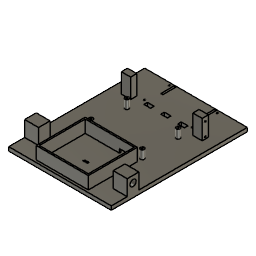
chassis (Autodesk Fusion 360 design; units mm, degrees)
part number: 2026-04-02-12-57-44-250
Autodesk Fusion 360 part; units mm, degrees
other "DerivedContext1"
sketch "Sketch1" plane through (0, 0, 0) normal (0, 0, 1) x (1, 0, 0)
  line L0 (0, 0) -> (132, 0)
  line L1 (132, 0) -> (132, 175)
  line L2 (132, 175) -> (0, 175)
  line L3 (0, 175) -> (0, 0)
  dimension "d1" = 132
  dimension "d2" = 175
  constraint horizontal L0
  constraint horizontal L2
  constraint coincident L0.start L3.end
  measures "d1" distance of L0.start L0.end
  measures "d2" distance of L0.end L1.end
extrude "Extrude1" add sketch "Sketch1" along normal blind 5
sketch "Sketch2" plane through (0, 0, 5) normal (0, 0, 1) x (-1, 0, 0)
  line L0 (0, -175) -> (0, 0)
  line L1 (0, 0) -> (-132, 0)
  line L2 (-132, 0) -> (-132, -175)
  line L3 (-132, -175) -> (0, -175)
  line L4 (-14, -175) -> (-14, -134.884) construction
  line L5 (-14, -134.884) -> (0, -134.884) construction
  line L6 (-14, -138.884) -> (-14, -130.884)
  line L7 (-14, -138.884) -> (-26, -138.884)
  line L8 (-26, -138.884) -> (-26, -130.884)
  line L9 (-14, -130.884) -> (-14, -138.884)
  line L10 (-14, -130.884) -> (-26, -130.884)
  line L11 (-66, -175) -> (-66, -165)
  line L12 (-118, -138.884) -> (-106, -138.884)
  line L13 (-106, -138.884) -> (-106, -130.884)
  line L14 (-118, -130.884) -> (-106, -130.884)
  line L15 (-118, -138.884) -> (-118, -130.884)
  dimension "d5" = 40.116
  dimension "d7" = 14
  dimension "d8" = 8
  dimension "d9" = 12
  dimension "d10" = 10
  constraint vertical L4
  constraint coincident L3 L4.start
  constraint coincident L0 L5.end
  constraint perpendicular L0 L5
  constraint vertical L6
  constraint midpoint L4.end L6
  constraint horizontal L7
  constraint vertical L8
  constraint vertical L9
  constraint perpendicular L8 L10
  constraint midpoint L3 L11.start
  constraint perpendicular L3 L11
  constraint symmetric L6.start L11 L12.start
  constraint symmetric L6.end L11 L14.start
  constraint symmetric L7.end L11 L12.end
  constraint symmetric L8.end L11 L13.end
  measures "d5" distance of L4.start L4.end
  measures "d7" distance of L4.end L5.end
  measures "d8" distance of L6.start L6.end
  measures "d9" distance of L6.start L7.end
  measures "d10" distance of L11.start L11.end
extrude "Extrude2" add sketch "Sketch2" along normal blind 25 contours L6 L7 L8 L9 L10 | L12 L13 L14 L15
ref_plane "WorkPlane1" through (66, 134.884, 17.5) normal (1, 0, 0) x (0, 1, 0)
sketch "Sketch4" plane through (0, 0, 5) normal (0, 0, 1) x (-1, 0, 0)
  line L0 (-106, -138.884) -> (-118, -138.884)
  line L1 (-118, -138.884) -> (-118, -130.884)
  line L2 (-118, -130.884) -> (-106, -130.884)
  line L3 (-106, -130.884) -> (-106, -138.884)
  line L4 (-14, -138.884) -> (-26, -138.884)
  line L5 (-26, -138.884) -> (-26, -130.884)
  line L6 (-26, -130.884) -> (-14, -130.884)
  line L7 (-14, -130.884) -> (-14, -138.884)
  line L8 (0, -175) -> (0, 0)
  line L9 (0, 0) -> (-132, 0)
  line L10 (-132, 0) -> (-132, -175)
  line L11 (-132, -175) -> (0, -175)
  line L12 (-41.25, -175) -> (-41.25, -157)
  line L13 (-41.25, -157) -> (-38.75, -157)
  line L14 (-38.75, -157) -> (-38.75, -175)
  dimension "d27" = 18
  dimension "d28" = 41.25
  dimension "d29" = 2.5
  constraint coincident L11 L12.start
  constraint perpendicular L11 L12
  constraint perpendicular L12 L13
  constraint vertical L14
  constraint coincident L11 L14.end
  measures "d27" distance of L12.start L12.end
  measures "d28" distance of L8 L12
  measures "d29" distance of L12.end L13.end
extrude "Extrude4" cut sketch "Sketch4" against normal blind 4 contours L11 L12 L13 L14
fillet "Fillet1" radius 4 1 edges at (40, 157, 1)
sketch "Sketch5" plane through (41.25, 0, 0) normal (-1, 0, 0) x (0, -1, 0)
  arc A0 (-161, 1) -> (-157, 5) centre (-161, 5) ccw
  line L0 (-157, 5) -> (-175, 5)
  line L1 (-175, 5) -> (-175, 1)
  line L2 (-175, 1) -> (-161, 1)
  line L3 (-175, 5) -> (-171, 5)
  circle A1 centre (-171, 5) radius 4
  dimension "d34" = 4
  dimension "d35" = 8
  constraint coincident L0.end L1.start
  constraint perpendicular L1 L3
  constraint coincident L3.end A1.centre
  measures "d34" distance of L0.end L3.end
  measures "d35" diameter of A1
extrude "Extrude5" add sketch "Sketch5" along normal blind 3 contours L1 L2 A1
ref_plane "WorkPlane3" through (66, 87.5, 2.5) normal (1, 0, 0) x (0, 1, 0)
mirror "Mirror2" about plane through (66, 87.5, 2.5) normal (1, 0, 0) of "Extrude4", "Fillet1", "Extrude5"
sketch "Battery Holder slot" plane through (0, 0, 5) normal (0, 0, 1) x (-1, 0, 0)
  line L0 (-14, -138.884) -> (-26, -138.884)
  line L1 (-26, -138.884) -> (-26, -130.884)
  line L2 (-26, -130.884) -> (-14, -130.884)
  line L3 (-14, -130.884) -> (-14, -138.884)
  line L4 (-106, -138.884) -> (-118, -138.884)
  line L5 (-118, -138.884) -> (-118, -130.884)
  line L6 (-118, -130.884) -> (-106, -130.884)
  line L7 (-106, -130.884) -> (-106, -138.884)
  line L8 (-93.25, -175) -> (-93.25, -157)
  line L9 (-93.25, -157) -> (-90.75, -157)
  line L10 (-90.75, -157) -> (-90.75, -175)
  line L11 (-90.75, -175) -> (-41.25, -175)
  line L12 (-41.25, -175) -> (-41.25, -157)
  line L13 (-41.25, -157) -> (-38.75, -157)
  line L14 (-38.75, -157) -> (-38.75, -175)
  line L15 (-38.75, -175) -> (0, -175)
  line L16 (0, -175) -> (0, 0)
  line L17 (0, 0) -> (-132, 0)
  line L18 (-132, 0) -> (-132, -175)
  line L19 (-132, -175) -> (-93.25, -175)
  line L20 (-34.5, -5) -> (-97.5, -5)
  line L21 (-97.5, -5) -> (-97.5, -64)
  line L22 (-97.5, -64) -> (-34.5, -64)
  line L23 (-34.5, -64) -> (-34.5, -5)
  line L24 (-66, 0) -> (-66, -5) construction
  line L25 (-32.5, -66) -> (-99.5, -66)
  line L26 (-99.5, -66) -> (-99.5, -3)
  line L27 (-99.5, -3) -> (-32.5, -3)
  line L28 (-32.5, -3) -> (-32.5, -66)
  dimension "d40" = 63
  dimension "d41" = 59
  dimension "d42" = 5
  dimension "d43" = 2
  dimension "d44" = 2
  dimension "d45" = 2
  dimension "d46" = 2
  constraint horizontal L20
  constraint vertical L21
  constraint horizontal L22
  constraint vertical L23
  constraint midpoint L17 L24.start
  constraint perpendicular L20 L24
  constraint coincident L20 L24.end
  constraint midpoint L20 L24.end
  constraint horizontal L25
  constraint vertical L26
  constraint horizontal L27
  constraint vertical L28
  measures "d40" distance of L20.start L20.end
  measures "d41" distance of L20.start L22.end
  measures "d42" distance of L17 L20
  measures "d43" distance of L23 L28
  measures "d44" distance of L22 L25
  measures "d45" distance of L21 L26
  measures "d46" distance of L20 L27
extrude "Extrude6" add sketch "Battery Holder slot" along normal blind 16 contours L25 L26 L27 L28
sketch "Battery Holder Hole" plane through (0, 66, 0) normal (0, 1, 0) x (-1, 0, 0)
  line L0 (-99.5, 5) -> (-32.5, 5)
  line L1 (-32.5, 5) -> (-32.5, 21)
  line L2 (-32.5, 21) -> (-99.5, 21)
  line L3 (-99.5, 21) -> (-99.5, 5)
  line L4 (-99.5, 5) -> (-78.5, 5)
  line L5 (-99.5, 5) -> (-88.5, 5)
  line L6 (-88.5, 5) -> (-78.5, 5)
  line L7 (-78.5, 5) -> (-78.5, 10)
  line L8 (-78.5, 10) -> (-88.5, 10)
  line L9 (-88.5, 10) -> (-88.5, 5)
  dimension "d50" = 11
  dimension "d51" = 10
  dimension "d52" = 5
  constraint coincident L0.start L3.end
  constraint perpendicular L3 L4
  constraint perpendicular L3 L5
  constraint horizontal L6
  constraint vertical L7
  constraint horizontal L8
  constraint vertical L9
  measures "d50" distance of L0.start L5.end
  measures "d51" distance of L5.end L4.end
  measures "d52" distance of L5.end L8.end
extrude "Extrude7" cut sketch "Battery Holder Hole" against normal blind 2 contours L0 L4 L6 L7 L8 L9
sketch "Rear Shaft Holder" plane through (0, 0, 5) normal (0, 0, 1) x (-1, 0, 0)
  line L0 (-14, -138.884) -> (-26, -138.884)
  line L1 (-26, -138.884) -> (-26, -130.884)
  line L2 (-26, -130.884) -> (-14, -130.884)
  line L3 (-14, -130.884) -> (-14, -138.884)
  line L4 (-106, -138.884) -> (-118, -138.884)
  line L5 (-118, -138.884) -> (-118, -130.884)
  line L6 (-118, -130.884) -> (-106, -130.884)
  line L7 (-106, -130.884) -> (-106, -138.884)
  line L8 (-93.25, -175) -> (-93.25, -157)
  line L9 (-93.25, -157) -> (-90.75, -157)
  line L10 (-90.75, -157) -> (-90.75, -175)
  line L11 (-90.75, -175) -> (-41.25, -175)
  line L12 (-41.25, -175) -> (-41.25, -157)
  line L13 (-41.25, -157) -> (-38.75, -157)
  line L14 (-38.75, -157) -> (-38.75, -175)
  line L15 (-38.75, -175) -> (0, -175)
  line L16 (0, -175) -> (0, 0)
  line L17 (0, 0) -> (-132, 0)
  line L18 (-132, 0) -> (-132, -175)
  line L19 (-132, -175) -> (-93.25, -175)
  line L20 (-34.5, -5) -> (-97.5, -5)
  line L21 (-97.5, -5) -> (-97.5, -64)
  line L22 (-97.5, -64) -> (-88.5, -64)
  line L23 (-88.5, -64) -> (-88.5, -66)
  line L24 (-88.5, -66) -> (-99.5, -66)
  line L25 (-99.5, -66) -> (-99.5, -3)
  line L26 (-99.5, -3) -> (-32.5, -3)
  line L27 (-32.5, -3) -> (-32.5, -66)
  line L28 (-32.5, -66) -> (-78.5, -66)
  line L29 (-78.5, -66) -> (-78.5, -64)
  line L30 (-78.5, -64) -> (-34.5, -64)
  line L31 (-34.5, -64) -> (-34.5, -5)
  line L32 (0, 0) -> (0, -28)
  line L33 (0, -35.5) -> (-18, -35.5)
  line L34 (-18, -35.5) -> (-18, -20.5)
  line L35 (-18, -20.5) -> (0, -20.5)
  line L36 (0, -20.5) -> (0, -35.5)
  dimension "d55" = 28
  dimension "d56" = 18
  dimension "d57" = 15
  constraint coincident L16.end L17.start
  constraint perpendicular L17 L32
  constraint horizontal L33
  constraint vertical L34
  constraint horizontal L35
  constraint vertical L36
  constraint coincident L16 L33.start
  constraint midpoint L32.end L36
  measures "d55" distance of L16.end L32.end
  measures "d56" distance of L33.start L33.end
  measures "d57" distance of L33.start L35.end
extrude "Extrude8" add sketch "Rear Shaft Holder" along normal blind 20 contours L16 L32 L33 L34 L35 L36
mirror "Mirror3" about plane through (66, 87.5, 2.5) normal (1, 0, 0) of "Extrude8"
sketch "Rear Shaft Hole" plane through (0, 0, 0) normal (-1, 0, 0) x (0, -1, 0)
  line L0 (-175, 0) -> (0, 0)
  line L1 (0, 0) -> (0, 5)
  line L2 (0, 5) -> (-20.5, 5)
  line L3 (-20.5, 5) -> (-20.5, 25)
  line L4 (-20.5, 25) -> (-35.5, 25)
  line L5 (-35.5, 25) -> (-35.5, 5)
  line L6 (-35.5, 5) -> (-175, 5)
  line L7 (-175, 5) -> (-175, 0)
  line L8 (-35.5, 5) -> (-20.5, 5)
  line L9 (-28, 5) -> (-28, 16.5)
  circle A0 centre (-28, 16.5) radius 4
  dimension "d62" = 11.5
  dimension "d63" = 8
  constraint coincident L5.end L6.start
  constraint coincident L2.end L3.start
  constraint midpoint L8 L9.start
  constraint perpendicular L8 L9
  constraint coincident L9.end A0.centre
  measures "d62" distance of L9.start L9.end
  measures "d63" diameter of A0
extrude "Extrude9" cut sketch "Rear Shaft Hole" against normal blind 14 contours A0
mirror "Mirror4" about plane through (66, 87.5, 2.5) normal (1, 0, 0) of "Extrude9"
sketch "Sketch11" plane through (0, 0, 5) normal (0, 0, 1) x (-1, 0, 0)
  line L0 (-14, -138.884) -> (-26, -138.884)
  line L1 (-26, -138.884) -> (-26, -130.884)
  line L2 (-26, -130.884) -> (-14, -130.884)
  line L3 (-14, -130.884) -> (-14, -138.884)
  line L4 (-106, -138.884) -> (-118, -138.884)
  line L5 (-118, -138.884) -> (-118, -130.884)
  line L6 (-118, -130.884) -> (-106, -130.884)
  line L7 (-106, -130.884) -> (-106, -138.884)
  line L8 (-132, -20.5) -> (-114, -20.5)
  line L9 (-114, -20.5) -> (-114, -35.5)
  line L10 (-114, -35.5) -> (-132, -35.5)
  line L11 (-132, -35.5) -> (-132, -175)
  line L12 (-132, -175) -> (-93.25, -175)
  line L13 (-93.25, -175) -> (-93.25, -157)
  line L14 (-93.25, -157) -> (-90.75, -157)
  line L15 (-90.75, -157) -> (-90.75, -175)
  line L16 (-90.75, -175) -> (-41.25, -175)
  line L17 (-41.25, -175) -> (-41.25, -157)
  line L18 (-41.25, -157) -> (-38.75, -157)
  line L19 (-38.75, -157) -> (-38.75, -175)
  line L20 (-38.75, -175) -> (0, -175)
  line L21 (0, -175) -> (0, -35.5)
  line L22 (0, -35.5) -> (-18, -35.5)
  line L23 (-18, -35.5) -> (-18, -20.5)
  line L24 (-18, -20.5) -> (0, -20.5)
  line L25 (0, -20.5) -> (0, 0)
  line L26 (0, 0) -> (-132, 0)
  line L27 (-132, 0) -> (-132, -20.5)
  line L28 (-34.5, -5) -> (-97.5, -5)
  line L29 (-97.5, -5) -> (-97.5, -64)
  line L30 (-97.5, -64) -> (-88.5, -64)
  line L31 (-88.5, -64) -> (-88.5, -66)
  line L32 (-88.5, -66) -> (-99.5, -66)
  line L33 (-99.5, -66) -> (-99.5, -3)
  line L34 (-99.5, -3) -> (-32.5, -3)
  line L35 (-32.5, -3) -> (-32.5, -66)
  line L36 (-32.5, -66) -> (-78.5, -66)
  line L37 (-78.5, -66) -> (-78.5, -64)
  line L38 (-78.5, -64) -> (-34.5, -64)
  line L39 (-34.5, -64) -> (-34.5, -5)
  line L40 (-101, -71) -> (-31, -71) construction
  line L41 (-31, -71) -> (-31, -121) construction
  line L42 (-31, -121) -> (-101, -121) construction
  line L43 (-101, -121) -> (-101, -71) construction
  line L44 (-99.5, -66) -> (-32.5, -66) construction
  line L45 (-66, -66) -> (-66, -71) construction
  line L46 (-101, -71) -> (-99, -71)
  line L47 (-99, -71) -> (-99, -73) construction
  line L48 (-99, -73) -> (-101, -73) construction
  line L49 (-101, -73) -> (-101, -71)
  circle A0 centre (-99, -73) radius 2.5
  circle A1 centre (-99, -73) radius 1
  line L50 (-101, -96) -> (-31, -96)
  circle A2 centre (-99, -119) radius 1
  circle A3 centre (-99, -119) radius 2.5
  line L51 (-66, -121) -> (-66, -71)
  circle A4 centre (-33, -119) radius 2.5
  circle A5 centre (-33, -119) radius 1
  circle A6 centre (-33, -73) radius 2.5
  circle A7 centre (-33, -73) radius 1
  dimension "d68" = 70
  dimension "d69" = 50
  dimension "d70" = 5
  dimension "d84" = 2
  dimension "d85" = 2
  dimension "d86" = 5
  dimension "d87" = 2
  constraint horizontal L40
  constraint vertical L41
  constraint horizontal L42
  constraint vertical L43
  constraint coincident L32.end L33.start
  constraint coincident L35.end L36.start
  constraint midpoint L44 L45.start
  constraint perpendicular L40 L45
  constraint midpoint L40 L45.end
  constraint horizontal L46
  constraint vertical L47
  constraint horizontal L48
  constraint vertical L49
  constraint coincident L47.end L48.start
  constraint midpoint L43 L50.start
  constraint midpoint L41 L50.end
  constraint symmetric A0 L50 A3
  constraint symmetric A1 L50 A2
  constraint midpoint L42 L51.start
  constraint symmetric A0 L51 A6
  constraint symmetric A1 L51 A7
  constraint symmetric A2 L51 A5
  constraint symmetric A3 L51 A4
  measures "d68" distance of L40.start L40.end
  measures "d69" distance of L40.start L42.end
  measures "d70" distance of L45.start L45.end
  measures "d84" distance of L40.start L46.end
  measures "d85" distance of L40.start L48.end
  measures "d86" diameter of A0
  measures "d87" diameter of A1
extrude "Extrude10" add sketch "Sketch11" along normal blind 11 contours A0 | A3 | A4 | A6
sketch "Sketch12" plane through (0, 0, 5) normal (0, 0, 1) x (-1, 0, 0)
  circle A0 centre (-99, -119) radius 2.5
  circle A1 centre (-33, -119) radius 2.5
  line L0 (-14, -138.884) -> (-26, -138.884)
  line L1 (-26, -138.884) -> (-26, -130.884)
  line L2 (-26, -130.884) -> (-14, -130.884)
  line L3 (-14, -130.884) -> (-14, -138.884)
  line L4 (-106, -138.884) -> (-118, -138.884)
  line L5 (-118, -138.884) -> (-118, -130.884)
  line L6 (-118, -130.884) -> (-106, -130.884)
  line L7 (-106, -130.884) -> (-106, -138.884)
  line L8 (-132, -20.5) -> (-114, -20.5)
  line L9 (-114, -20.5) -> (-114, -35.5)
  line L10 (-114, -35.5) -> (-132, -35.5)
  line L11 (-132, -35.5) -> (-132, -175)
  line L12 (-132, -175) -> (-93.25, -175)
  line L13 (-93.25, -175) -> (-93.25, -157)
  line L14 (-93.25, -157) -> (-90.75, -157)
  line L15 (-90.75, -157) -> (-90.75, -175)
  line L16 (-90.75, -175) -> (-41.25, -175)
  line L17 (-41.25, -175) -> (-41.25, -157)
  line L18 (-41.25, -157) -> (-38.75, -157)
  line L19 (-38.75, -157) -> (-38.75, -175)
  line L20 (-38.75, -175) -> (0, -175)
  line L21 (0, -175) -> (0, -35.5)
  line L22 (0, -35.5) -> (-18, -35.5)
  line L23 (-18, -35.5) -> (-18, -20.5)
  line L24 (-18, -20.5) -> (0, -20.5)
  line L25 (0, -20.5) -> (0, 0)
  line L26 (0, 0) -> (-132, 0)
  line L27 (-132, 0) -> (-132, -20.5)
  line L28 (-34.5, -5) -> (-97.5, -5)
  line L29 (-97.5, -5) -> (-97.5, -64)
  line L30 (-97.5, -64) -> (-88.5, -64)
  line L31 (-88.5, -64) -> (-88.5, -66)
  line L32 (-88.5, -66) -> (-99.5, -66)
  line L33 (-99.5, -66) -> (-99.5, -3)
  line L34 (-99.5, -3) -> (-32.5, -3)
  line L35 (-32.5, -3) -> (-32.5, -66)
  line L36 (-32.5, -66) -> (-78.5, -66)
  line L37 (-78.5, -66) -> (-78.5, -64)
  line L38 (-78.5, -64) -> (-34.5, -64)
  line L39 (-34.5, -64) -> (-34.5, -5)
  circle A2 centre (-33, -73) radius 2.5
  circle A3 centre (-99, -73) radius 2.5
  line L40 (-68.991, -34.5196) -> (-63.009, -34.4804) construction
  line L41 (-63.009, -34.4804) -> (-63.0241, -32.1688) construction
  line L42 (-63.0241, -32.1688) -> (-69.0062, -32.208) construction
  line L43 (-69.0062, -32.208) -> (-68.991, -34.5196) construction
  line L44 (-97.5, -34.5) -> (-34.5, -34.5)
  line L45 (-66, -5) -> (-66, -34.5)
  dimension "d90" = 2
  text T0 "BAT" font "Arial Black" height 2 align left top in box 5.9822 x 2.3117 at (-68.991, -34.5196) x (0.999979, 0.006542) y (-0.006542, 0.999979) spacing 1.01 kerned
  constraint midpoint L29 L44.start
  constraint midpoint L39 L44.end
  constraint midpoint L28 L45.start
  constraint midpoint L44 L45.end
extrude "Extrude11" cut sketch "Sketch12" against normal blind 0.5 text T0
move_body "Move2" bodies 1 to x (1, 0, 0) y (0, 1, 0) z (0, 0, 1) at (0, 0, 21.4)
sketch "Sketch15" plane through (0, 0, 26.4) normal (0, 0, 1) x (-1, 0, 0)
  circle A0 centre (-99, -73) radius 2.5
  circle A1 centre (-33, -73) radius 2.5
  line L0 (-34.5, -5) -> (-97.5, -5)
  line L1 (-97.5, -5) -> (-97.5, -64)
  line L2 (-97.5, -64) -> (-88.5, -64)
  line L3 (-88.5, -64) -> (-88.5, -66)
  line L4 (-88.5, -66) -> (-99.5, -66)
  line L5 (-99.5, -66) -> (-99.5, -3)
  line L6 (-99.5, -3) -> (-32.5, -3)
  line L7 (-32.5, -3) -> (-32.5, -66)
  line L8 (-32.5, -66) -> (-78.5, -66)
  line L9 (-78.5, -66) -> (-78.5, -64)
  line L10 (-78.5, -64) -> (-34.5, -64)
  line L11 (-34.5, -64) -> (-34.5, -5)
  line L12 (-132, -20.5) -> (-114, -20.5)
  line L13 (-114, -20.5) -> (-114, -35.5)
  line L14 (-114, -35.5) -> (-132, -35.5)
  line L15 (-132, -35.5) -> (-132, -175)
  line L16 (-132, -175) -> (-93.25, -175)
  line L17 (-93.25, -175) -> (-93.25, -157)
  line L18 (-93.25, -157) -> (-90.75, -157)
  line L19 (-90.75, -157) -> (-90.75, -175)
  line L20 (-90.75, -175) -> (-41.25, -175)
  line L21 (-41.25, -175) -> (-41.25, -157)
  line L22 (-41.25, -157) -> (-38.75, -157)
  line L23 (-38.75, -157) -> (-38.75, -175)
  line L24 (-38.75, -175) -> (0, -175)
  line L25 (0, -175) -> (0, -35.5)
  line L26 (0, -35.5) -> (-18, -35.5)
  line L27 (-18, -35.5) -> (-18, -20.5)
  line L28 (-18, -20.5) -> (0, -20.5)
  line L29 (0, -20.5) -> (0, 0)
  line L30 (0, 0) -> (-132, 0)
  line L31 (-132, 0) -> (-132, -20.5)
  line L32 (-106, -138.884) -> (-118, -138.884)
  line L33 (-118, -138.884) -> (-118, -130.884)
  line L34 (-118, -130.884) -> (-106, -130.884)
  line L35 (-106, -130.884) -> (-106, -138.884)
  line L36 (-14, -138.884) -> (-26, -138.884)
  line L37 (-26, -138.884) -> (-26, -130.884)
  line L38 (-26, -130.884) -> (-14, -130.884)
  line L39 (-14, -130.884) -> (-14, -138.884)
  circle A2 centre (-33, -119) radius 2.5
  circle A3 centre (-99, -119) radius 2.5
  line L40 (-67.9262, -34.2009) -> (-68.9931, -34.2079)
  line L41 (-68.9931, -34.2079) -> (-69.0062, -32.208)
  line L42 (-69.0062, -32.208) -> (-67.8493, -32.2004)
  spline S0 degree 3 poles (-67.8493, -32.2004) (-67.7612, -32.2034) (-67.5991, -32.209) (-67.4654, -32.2994) (-67.4043, -32.3407) knots 0 0 0 0 0.025812 0.047504 0.047504 0.047504 0.047504
  spline S1 degree 3 poles (-67.4043, -32.3407) (-67.3588, -32.391) (-67.2678, -32.4917) (-67.254, -32.6268) (-67.2471, -32.6944) knots 0 0 0 0 0.019795 0.039617 0.039617 0.039617 0.039617
  spline S2 degree 3 poles (-67.2471, -32.6944) (-67.2511, -32.7511) (-67.2589, -32.863) (-67.3237, -32.9543) (-67.3556, -32.9994) knots 0 0 0 0 0.016703 0.032929 0.032929 0.032929 0.032929
  spline S3 degree 3 poles (-67.3556, -32.9994) (-67.3844, -33.0268) (-67.4468, -33.0861) (-67.5271, -33.1176) (-67.5703, -33.1345) knots 0 0 0 0 0.011817 0.025581 0.025581 0.025581 0.025581
  spline S4 degree 3 poles (-67.5703, -33.1345) (-67.5049, -33.1524) (-67.3841, -33.1854) (-67.2935, -33.2711) (-67.252, -33.3104) knots 0 0 0 0 0.019989 0.036874 0.036874 0.036874 0.036874
  spline S5 degree 3 poles (-67.252, -33.3104) (-67.222, -33.3563) (-67.1594, -33.4524) (-67.1521, -33.567) (-67.1483, -33.6269) knots 0 0 0 0 0.016151 0.033815 0.033815 0.033815 0.033815
  spline S6 degree 3 poles (-67.1483, -33.6269) (-67.1507, -33.677) (-67.1554, -33.7752) (-67.1979, -33.8637) (-67.2187, -33.9071) knots 0 0 0 0 0.014878 0.029148 0.029148 0.029148 0.029148
  spline S7 degree 3 poles (-67.2187, -33.9071) (-67.2448, -33.9465) (-67.2972, -34.0255) (-67.3758, -34.0783) (-67.4153, -34.1048) knots 0 0 0 0 0.014032 0.028126 0.028126 0.028126 0.028126
  spline S8 degree 3 poles (-67.4153, -34.1048) (-67.4473, -34.1193) (-67.5219, -34.1532) (-67.6031, -34.165) (-67.6495, -34.1718) knots 0 0 0 0 0.010501 0.024467 0.024467 0.024467 0.024467
  spline S9 degree 3 poles (-67.6495, -34.1718) (-67.7072, -34.18) (-67.7991, -34.1929) (-67.8918, -34.1988) (-67.9262, -34.2009) knots 0 0 0 0 0.01748 0.027837 0.027837 0.027837 0.027837
  line L43 (-64.8768, -34.181) -> (-65.5239, -34.1852)
  line L44 (-65.5239, -34.1852) -> (-65.6261, -33.8557)
  line L45 (-65.6261, -33.8557) -> (-66.3277, -33.8603)
  line L46 (-66.3277, -33.8603) -> (-66.4231, -34.1911)
  line L47 (-66.4231, -34.1911) -> (-67.0541, -34.1952)
  line L48 (-67.0541, -34.1952) -> (-66.3155, -32.1903)
  line L49 (-66.3155, -32.1903) -> (-65.6414, -32.1859)
  line L50 (-65.6414, -32.1859) -> (-64.8768, -34.181)
  line L51 (-64.3773, -32.6715) -> (-65.0076, -32.6757)
  line L52 (-65.0076, -32.6757) -> (-65.0108, -32.1818)
  line L53 (-65.0108, -32.1818) -> (-63.1323, -32.1695)
  line L54 (-63.1323, -32.1695) -> (-63.1291, -32.6634)
  line L55 (-63.1291, -32.6634) -> (-63.7593, -32.6675)
  line L56 (-63.7593, -32.6675) -> (-63.7495, -34.1736)
  line L57 (-63.7495, -34.1736) -> (-64.3675, -34.1776)
  line L58 (-64.3675, -34.1776) -> (-64.3773, -32.6715)
  line L59 (-92, -119) -> (-40, -119)
  line L60 (-92, -119) -> (-92, -134)
  line L61 (-40, -119) -> (-40, -134)
  line L62 (-92, -134) -> (-40, -134)
  line L63 (-92, -134) -> (-83.5, -134)
  line L64 (-83.5, -134) -> (-83.5, -138.5)
  line L65 (-83.5, -138.5) -> (-92, -138.5)
  line L66 (-92, -138.5) -> (-92, -134)
  line L67 (-66, -134) -> (-66, -138.5) construction
  line L68 (-70.25, -138.5) -> (-61.75, -138.5)
  line L69 (-70.25, -138.5) -> (-70.25, -134)
  line L70 (-61.75, -138.5) -> (-61.75, -134)
  line L71 (-92, -134) -> (-83.5, -134)
  line L72 (-40, -134) -> (-48.5, -134)
  line L73 (-48.5, -134) -> (-48.5, -138.5)
  line L74 (-48.5, -138.5) -> (-40, -138.5)
  line L75 (-40, -138.5) -> (-40, -134)
  line L76 (-99, -119) -> (-92, -119)
  line L77 (-33, -119) -> (-40, -119)
  dimension "d94" = 15
  dimension "d96" = 8.5
  dimension "d97" = 4.5
  dimension "d98" = 4.5
  dimension "d99" = 8.5
  dimension "d102" = 52
  constraint horizontal L59
  constraint perpendicular L59 L60
  constraint perpendicular L59 L61
  constraint horizontal L63
  constraint vertical L64
  constraint horizontal L65
  constraint vertical L66
  constraint midpoint L62 L67.start
  constraint perpendicular L62 L67
  constraint horizontal L68
  constraint midpoint L67.end L68
  constraint coincident L62 L69.end
  constraint perpendicular L62 L69
  constraint coincident L62 L70.end
  constraint perpendicular L62 L70
  constraint symmetric L60.end L67 L61.end
  constraint symmetric L63.end L67 L72.end
  constraint symmetric L64.end L67 L73.end
  constraint symmetric L65.end L67 L74.end
  constraint coincident L59.end L61.start
  constraint coincident L59.start L60.start
  constraint perpendicular L61 L62
  constraint coincident A3.centre L76.start
  constraint coincident A2.centre L77.start
  constraint parallel L59 L77
  constraint equal L76 L77
  measures "d94" distance of L59.start L60.end
  measures "d96" distance of L60.end L63.end
  measures "d97" distance of L60.end L65.end
  measures "d98" distance of L67.start L67.end
  measures "d99" distance of L68.start L68.end
  measures "d102" distance of L59.start L59.end
extrude "Extrude12" cut sketch "Sketch15" against normal blind 5 contours L62 L63 L64 L65 L66 L71 | L62 L72 L73 L74 L75 | L62 L68 L69 L70
sketch "Sketch16" plane through (0, 0, 21.4) normal (0, 0, -1) x (1, 0, 0)
  line L0 (61.75, -138.5) -> (61.75, -134)
  line L1 (61.75, -134) -> (70.25, -134)
  line L2 (70.25, -134) -> (70.25, -138.5)
  line L3 (70.25, -138.5) -> (61.75, -138.5)
  line L4 (92, -138.5) -> (83.5, -138.5)
  line L5 (83.5, -138.5) -> (83.5, -134)
  line L6 (83.5, -134) -> (92, -134)
  line L7 (92, -134) -> (92, -138.5)
  line L8 (40, -134) -> (48.5, -134)
  line L9 (48.5, -134) -> (48.5, -138.5)
  line L10 (48.5, -138.5) -> (40, -138.5)
  line L11 (40, -138.5) -> (40, -134)
  line L12 (0, 0) -> (0, -175)
  line L13 (0, -175) -> (132, -175)
  line L14 (132, -175) -> (132, 0)
  line L15 (132, 0) -> (0, 0)
sketch "Sketch17" plane through (0, 0, 26.4) normal (0, 0, 1) x (-1, 0, 0)
  line L0 (-61.75, -134) -> (-61.75, -138.5)
  line L1 (-61.75, -138.5) -> (-70.25, -138.5)
  line L2 (-70.25, -138.5) -> (-70.25, -134)
  line L3 (-70.25, -134) -> (-61.75, -134)
  line L4 (-83.5, -138.5) -> (-92, -138.5)
  line L5 (-92, -138.5) -> (-92, -134)
  line L6 (-92, -134) -> (-83.5, -134)
  line L7 (-83.5, -134) -> (-83.5, -138.5)
  line L8 (-48.5, -134) -> (-40, -134)
  line L9 (-40, -134) -> (-40, -138.5)
  line L10 (-40, -138.5) -> (-48.5, -138.5)
  line L11 (-48.5, -138.5) -> (-48.5, -134)
  circle A0 centre (-99, -73) radius 2.5
  circle A1 centre (-33, -73) radius 2.5
  line L12 (-34.5, -5) -> (-97.5, -5)
  line L13 (-97.5, -5) -> (-97.5, -64)
  line L14 (-97.5, -64) -> (-88.5, -64)
  line L15 (-88.5, -64) -> (-88.5, -66)
  line L16 (-88.5, -66) -> (-99.5, -66)
  line L17 (-99.5, -66) -> (-99.5, -3)
  line L18 (-99.5, -3) -> (-32.5, -3)
  line L19 (-32.5, -3) -> (-32.5, -66)
  line L20 (-32.5, -66) -> (-78.5, -66)
  line L21 (-78.5, -66) -> (-78.5, -64)
  line L22 (-78.5, -64) -> (-34.5, -64)
  line L23 (-34.5, -64) -> (-34.5, -5)
  line L24 (-132, -20.5) -> (-114, -20.5)
  line L25 (-114, -20.5) -> (-114, -35.5)
  line L26 (-114, -35.5) -> (-132, -35.5)
  line L27 (-132, -35.5) -> (-132, -175)
  line L28 (-132, -175) -> (-93.25, -175)
  line L29 (-93.25, -175) -> (-93.25, -157)
  line L30 (-93.25, -157) -> (-90.75, -157)
  line L31 (-90.75, -157) -> (-90.75, -175)
  line L32 (-90.75, -175) -> (-41.25, -175)
  line L33 (-41.25, -175) -> (-41.25, -157)
  line L34 (-41.25, -157) -> (-38.75, -157)
  line L35 (-38.75, -157) -> (-38.75, -175)
  line L36 (-38.75, -175) -> (0, -175)
  line L37 (0, -175) -> (0, -35.5)
  line L38 (0, -35.5) -> (-18, -35.5)
  line L39 (-18, -35.5) -> (-18, -20.5)
  line L40 (-18, -20.5) -> (0, -20.5)
  line L41 (0, -20.5) -> (0, 0)
  line L42 (0, 0) -> (-132, 0)
  line L43 (-132, 0) -> (-132, -20.5)
  line L44 (-106, -138.884) -> (-118, -138.884)
  line L45 (-118, -138.884) -> (-118, -130.884)
  line L46 (-118, -130.884) -> (-106, -130.884)
  line L47 (-106, -130.884) -> (-106, -138.884)
  line L48 (-14, -138.884) -> (-26, -138.884)
  line L49 (-26, -138.884) -> (-26, -130.884)
  line L50 (-26, -130.884) -> (-14, -130.884)
  line L51 (-14, -130.884) -> (-14, -138.884)
  circle A2 centre (-33, -119) radius 2.5
  circle A3 centre (-99, -119) radius 2.5
  line L52 (-67.9262, -34.2009) -> (-68.9931, -34.2079)
  line L53 (-68.9931, -34.2079) -> (-69.0062, -32.208)
  line L54 (-69.0062, -32.208) -> (-67.8493, -32.2004)
  spline S0 degree 3 poles (-67.8493, -32.2004) (-67.7612, -32.2034) (-67.5991, -32.209) (-67.4654, -32.2994) (-67.4043, -32.3407) knots 0 0 0 0 0.025812 0.047504 0.047504 0.047504 0.047504
  spline S1 degree 3 poles (-67.4043, -32.3407) (-67.3588, -32.391) (-67.2678, -32.4917) (-67.254, -32.6268) (-67.2471, -32.6944) knots 0 0 0 0 0.019795 0.039617 0.039617 0.039617 0.039617
  spline S2 degree 3 poles (-67.2471, -32.6944) (-67.2511, -32.7511) (-67.2589, -32.863) (-67.3237, -32.9543) (-67.3556, -32.9994) knots 0 0 0 0 0.016703 0.032929 0.032929 0.032929 0.032929
  spline S3 degree 3 poles (-67.3556, -32.9994) (-67.3844, -33.0268) (-67.4468, -33.0861) (-67.5271, -33.1176) (-67.5703, -33.1345) knots 0 0 0 0 0.011817 0.025581 0.025581 0.025581 0.025581
  spline S4 degree 3 poles (-67.5703, -33.1345) (-67.5049, -33.1524) (-67.3841, -33.1854) (-67.2935, -33.2711) (-67.252, -33.3104) knots 0 0 0 0 0.019989 0.036874 0.036874 0.036874 0.036874
  spline S5 degree 3 poles (-67.252, -33.3104) (-67.222, -33.3563) (-67.1594, -33.4524) (-67.1521, -33.567) (-67.1483, -33.6269) knots 0 0 0 0 0.016151 0.033815 0.033815 0.033815 0.033815
  spline S6 degree 3 poles (-67.1483, -33.6269) (-67.1507, -33.677) (-67.1554, -33.7752) (-67.1979, -33.8637) (-67.2187, -33.9071) knots 0 0 0 0 0.014878 0.029148 0.029148 0.029148 0.029148
  spline S7 degree 3 poles (-67.2187, -33.9071) (-67.2448, -33.9465) (-67.2972, -34.0255) (-67.3758, -34.0783) (-67.4153, -34.1048) knots 0 0 0 0 0.014032 0.028126 0.028126 0.028126 0.028126
  spline S8 degree 3 poles (-67.4153, -34.1048) (-67.4473, -34.1193) (-67.5219, -34.1532) (-67.6031, -34.165) (-67.6495, -34.1718) knots 0 0 0 0 0.010501 0.024467 0.024467 0.024467 0.024467
  spline S9 degree 3 poles (-67.6495, -34.1718) (-67.7072, -34.18) (-67.7991, -34.1929) (-67.8918, -34.1988) (-67.9262, -34.2009) knots 0 0 0 0 0.01748 0.027837 0.027837 0.027837 0.027837
  line L55 (-64.8768, -34.181) -> (-65.5239, -34.1852)
  line L56 (-65.5239, -34.1852) -> (-65.6261, -33.8557)
  line L57 (-65.6261, -33.8557) -> (-66.3277, -33.8603)
  line L58 (-66.3277, -33.8603) -> (-66.4231, -34.1911)
  line L59 (-66.4231, -34.1911) -> (-67.0541, -34.1952)
  line L60 (-67.0541, -34.1952) -> (-66.3155, -32.1903)
  line L61 (-66.3155, -32.1903) -> (-65.6414, -32.1859)
  line L62 (-65.6414, -32.1859) -> (-64.8768, -34.181)
  line L63 (-64.3773, -32.6715) -> (-65.0076, -32.6757)
  line L64 (-65.0076, -32.6757) -> (-65.0108, -32.1818)
  line L65 (-65.0108, -32.1818) -> (-63.1323, -32.1695)
  line L66 (-63.1323, -32.1695) -> (-63.1291, -32.6634)
  line L67 (-63.1291, -32.6634) -> (-63.7593, -32.6675)
  line L68 (-63.7593, -32.6675) -> (-63.7495, -34.1736)
  line L69 (-63.7495, -34.1736) -> (-64.3675, -34.1776)
  line L70 (-64.3675, -34.1776) -> (-64.3773, -32.6715)
  line L71 (-87.75, -134) -> (-87.75, -138.5)
  line L72 (-66, -134) -> (-66, -138.5)
  line L73 (-66, -136.25) -> (-87.75, -136.25)
  constraint midpoint L6 L71.start
  constraint midpoint L4 L71.end
  constraint midpoint L3 L72.start
  constraint midpoint L1 L72.end
  constraint midpoint L72 L73.start
  constraint midpoint L71 L73.end
sketch "Sketch18" plane through (0, 0, 26.4) normal (0, 0, 1) x (-1, 0, 0)
  line L0 (-61.75, -134) -> (-61.75, -138.5)
  line L1 (-61.75, -138.5) -> (-70.25, -138.5)
  line L2 (-70.25, -138.5) -> (-70.25, -134)
  line L3 (-70.25, -134) -> (-61.75, -134)
  line L4 (-83.5, -138.5) -> (-92, -138.5)
  line L5 (-92, -138.5) -> (-92, -134)
  line L6 (-92, -134) -> (-83.5, -134)
  line L7 (-83.5, -134) -> (-83.5, -138.5)
  line L8 (-48.5, -134) -> (-40, -134)
  line L9 (-40, -134) -> (-40, -138.5)
  line L10 (-40, -138.5) -> (-48.5, -138.5)
  line L11 (-48.5, -138.5) -> (-48.5, -134)
  circle A0 centre (-99, -73) radius 2.5
  circle A1 centre (-33, -73) radius 2.5
  line L12 (-34.5, -5) -> (-97.5, -5)
  line L13 (-97.5, -5) -> (-97.5, -64)
  line L14 (-97.5, -64) -> (-88.5, -64)
  line L15 (-88.5, -64) -> (-88.5, -66)
  line L16 (-88.5, -66) -> (-99.5, -66)
  line L17 (-99.5, -66) -> (-99.5, -3)
  line L18 (-99.5, -3) -> (-32.5, -3)
  line L19 (-32.5, -3) -> (-32.5, -66)
  line L20 (-32.5, -66) -> (-78.5, -66)
  line L21 (-78.5, -66) -> (-78.5, -64)
  line L22 (-78.5, -64) -> (-34.5, -64)
  line L23 (-34.5, -64) -> (-34.5, -5)
  line L24 (-132, -20.5) -> (-114, -20.5)
  line L25 (-114, -20.5) -> (-114, -35.5)
  line L26 (-114, -35.5) -> (-132, -35.5)
  line L27 (-132, -35.5) -> (-132, -175)
  line L28 (-132, -175) -> (-93.25, -175)
  line L29 (-93.25, -175) -> (-93.25, -157)
  line L30 (-93.25, -157) -> (-90.75, -157)
  line L31 (-90.75, -157) -> (-90.75, -175)
  line L32 (-90.75, -175) -> (-41.25, -175)
  line L33 (-41.25, -175) -> (-41.25, -157)
  line L34 (-41.25, -157) -> (-38.75, -157)
  line L35 (-38.75, -157) -> (-38.75, -175)
  line L36 (-38.75, -175) -> (0, -175)
  line L37 (0, -175) -> (0, -35.5)
  line L38 (0, -35.5) -> (-18, -35.5)
  line L39 (-18, -35.5) -> (-18, -20.5)
  line L40 (-18, -20.5) -> (0, -20.5)
  line L41 (0, -20.5) -> (0, 0)
  line L42 (0, 0) -> (-132, 0)
  line L43 (-132, 0) -> (-132, -20.5)
  line L44 (-106, -138.884) -> (-118, -138.884)
  line L45 (-118, -138.884) -> (-118, -130.884)
  line L46 (-118, -130.884) -> (-106, -130.884)
  line L47 (-106, -130.884) -> (-106, -138.884)
  line L48 (-14, -138.884) -> (-26, -138.884)
  line L49 (-26, -138.884) -> (-26, -130.884)
  line L50 (-26, -130.884) -> (-14, -130.884)
  line L51 (-14, -130.884) -> (-14, -138.884)
  circle A2 centre (-33, -119) radius 2.5
  circle A3 centre (-99, -119) radius 2.5
  line L52 (-67.9262, -34.2009) -> (-68.9931, -34.2079)
  line L53 (-68.9931, -34.2079) -> (-69.0062, -32.208)
  line L54 (-69.0062, -32.208) -> (-67.8493, -32.2004)
  spline S0 degree 3 poles (-67.8493, -32.2004) (-67.7612, -32.2034) (-67.5991, -32.209) (-67.4654, -32.2994) (-67.4043, -32.3407) knots 0 0 0 0 0.025812 0.047504 0.047504 0.047504 0.047504
  spline S1 degree 3 poles (-67.4043, -32.3407) (-67.3588, -32.391) (-67.2678, -32.4917) (-67.254, -32.6268) (-67.2471, -32.6944) knots 0 0 0 0 0.019795 0.039617 0.039617 0.039617 0.039617
  spline S2 degree 3 poles (-67.2471, -32.6944) (-67.2511, -32.7511) (-67.2589, -32.863) (-67.3237, -32.9543) (-67.3556, -32.9994) knots 0 0 0 0 0.016703 0.032929 0.032929 0.032929 0.032929
  spline S3 degree 3 poles (-67.3556, -32.9994) (-67.3844, -33.0268) (-67.4468, -33.0861) (-67.5271, -33.1176) (-67.5703, -33.1345) knots 0 0 0 0 0.011817 0.025581 0.025581 0.025581 0.025581
  spline S4 degree 3 poles (-67.5703, -33.1345) (-67.5049, -33.1524) (-67.3841, -33.1854) (-67.2935, -33.2711) (-67.252, -33.3104) knots 0 0 0 0 0.019989 0.036874 0.036874 0.036874 0.036874
  spline S5 degree 3 poles (-67.252, -33.3104) (-67.222, -33.3563) (-67.1594, -33.4524) (-67.1521, -33.567) (-67.1483, -33.6269) knots 0 0 0 0 0.016151 0.033815 0.033815 0.033815 0.033815
  spline S6 degree 3 poles (-67.1483, -33.6269) (-67.1507, -33.677) (-67.1554, -33.7752) (-67.1979, -33.8637) (-67.2187, -33.9071) knots 0 0 0 0 0.014878 0.029148 0.029148 0.029148 0.029148
  spline S7 degree 3 poles (-67.2187, -33.9071) (-67.2448, -33.9465) (-67.2972, -34.0255) (-67.3758, -34.0783) (-67.4153, -34.1048) knots 0 0 0 0 0.014032 0.028126 0.028126 0.028126 0.028126
  spline S8 degree 3 poles (-67.4153, -34.1048) (-67.4473, -34.1193) (-67.5219, -34.1532) (-67.6031, -34.165) (-67.6495, -34.1718) knots 0 0 0 0 0.010501 0.024467 0.024467 0.024467 0.024467
  spline S9 degree 3 poles (-67.6495, -34.1718) (-67.7072, -34.18) (-67.7991, -34.1929) (-67.8918, -34.1988) (-67.9262, -34.2009) knots 0 0 0 0 0.01748 0.027837 0.027837 0.027837 0.027837
  line L55 (-64.8768, -34.181) -> (-65.5239, -34.1852)
  line L56 (-65.5239, -34.1852) -> (-65.6261, -33.8557)
  line L57 (-65.6261, -33.8557) -> (-66.3277, -33.8603)
  line L58 (-66.3277, -33.8603) -> (-66.4231, -34.1911)
  line L59 (-66.4231, -34.1911) -> (-67.0541, -34.1952)
  line L60 (-67.0541, -34.1952) -> (-66.3155, -32.1903)
  line L61 (-66.3155, -32.1903) -> (-65.6414, -32.1859)
  line L62 (-65.6414, -32.1859) -> (-64.8768, -34.181)
  line L63 (-64.3773, -32.6715) -> (-65.0076, -32.6757)
  line L64 (-65.0076, -32.6757) -> (-65.0108, -32.1818)
  line L65 (-65.0108, -32.1818) -> (-63.1323, -32.1695)
  line L66 (-63.1323, -32.1695) -> (-63.1291, -32.6634)
  line L67 (-63.1291, -32.6634) -> (-63.7593, -32.6675)
  line L68 (-63.7593, -32.6675) -> (-63.7495, -34.1736)
  line L69 (-63.7495, -34.1736) -> (-64.3675, -34.1776)
  line L70 (-64.3675, -34.1776) -> (-64.3773, -32.6715)
  line L71 (-66, -134) -> (-66, -138.5) construction
  line L72 (-70.25, -136.25) -> (-61.75, -136.25) construction
  circle A4 centre (-66, -136.25) radius 1
  dimension "d105" = 2
  constraint midpoint L3 L71.start
  constraint midpoint L1 L71.end
  constraint midpoint L2 L72.start
  constraint midpoint L0 L72.end
  constraint midpoint L72 A4.centre
  measures "d105" diameter of A4
sketch "Sketch19" plane through (0, 0, 21.4) normal (0, 0, -1) x (1, 0, 0)
  line L0 (61.75, -138.5) -> (61.75, -134)
  line L1 (61.75, -134) -> (70.25, -134)
  line L2 (70.25, -134) -> (70.25, -138.5)
  line L3 (70.25, -138.5) -> (61.75, -138.5)
  line L4 (92, -138.5) -> (83.5, -138.5)
  line L5 (83.5, -138.5) -> (83.5, -134)
  line L6 (83.5, -134) -> (92, -134)
  line L7 (92, -134) -> (92, -138.5)
  line L8 (40, -134) -> (48.5, -134)
  line L9 (48.5, -134) -> (48.5, -138.5)
  line L10 (48.5, -138.5) -> (40, -138.5)
  line L11 (40, -138.5) -> (40, -134)
  line L12 (0, 0) -> (0, -175)
  line L13 (0, -175) -> (132, -175)
  line L14 (132, -175) -> (132, 0)
  line L15 (132, 0) -> (0, 0)
  circle A0 centre (35.25, -171.45) radius 1
  circle A1 centre (35.25, -139.45) radius 1
  circle A2 centre (96.75, -139.45) radius 1
  circle A3 centre (96.75, -171.45) radius 1
  circle A4 centre (96.75, -171.45) radius 1
  circle A5 centre (35.25, -171.45) radius 1
  circle A6 centre (96.75, -139.45) radius 1
  circle A7 centre (35.25, -139.45) radius 1
  point P0 (96.75, -171.45)
  constraint coincident P0 A3.centre
  constraint concentric A0 A5
  constraint concentric A2 A6
  constraint concentric A1 A7
sketch "sketch 9845" plane through (96.75, 171.45, 16.4) normal (0, 0, -1) x (-1, 0, 0)
  line L0 (26.55, -25.2) -> (34.95, -25.2)
  line L1 (34.95, -25.2) -> (34.95, -29.2)
  line L2 (34.95, -29.2) -> (26.55, -29.2)
  line L3 (26.55, -29.2) -> (26.55, -25.2)
  line L4 (56.7, -25.2) -> (56.7, -29.2)
  line L5 (56.7, -29.2) -> (48.3, -29.2)
  line L6 (48.3, -29.2) -> (48.3, -25.2)
  line L7 (48.3, -25.2) -> (56.7, -25.2)
  line L8 (4.8, -29.2) -> (4.8, -25.2)
  line L9 (4.8, -25.2) -> (13.2, -25.2)
  line L10 (13.2, -25.2) -> (13.2, -29.2)
  line L11 (13.2, -29.2) -> (4.8, -29.2)
  line L12 (16.2, -9.3) -> (16.2, -16.8)
  line L13 (16.2, -16.8) -> (8.7, -16.8)
  line L14 (8.7, -16.8) -> (8.7, -9.3)
  line L15 (8.7, -9.3) -> (16.2, -9.3)
  line L16 (1.8, -1.8) -> (1.8, 1.8)
  arc A0 (1.8, 1.8) -> (0, -2.5456) centre (0, 0) ccw
  line L17 (0, -2.5456) -> (0, -29.4544)
  arc A1 (0, -29.4544) -> (2.5456, -32) centre (0, -32) ccw
  line L18 (2.5456, -32) -> (58.9544, -32)
  arc A2 (58.9544, -32) -> (61.5, -29.4544) centre (61.5, -32) ccw
  line L19 (61.5, -29.4544) -> (61.5, -2.5456)
  arc A3 (61.5, -2.5456) -> (59.6731, 1.7727) centre (61.5, 0) ccw
  line L20 (59.6731, 1.7727) -> (59.6731, -1.7727)
  arc A4 (59.6731, -1.7727) -> (59.7, -1.8) centre (61.5, 0) ccw
  line L21 (59.7, -1.8) -> (45.3, -1.8)
  line L22 (45.3, -1.8) -> (45.3, 1.8)
  line L23 (45.3, 1.8) -> (37.95, 1.8)
  line L24 (37.95, 1.8) -> (37.95, -1.8)
  line L25 (37.95, -1.8) -> (23.55, -1.8)
  line L26 (23.55, -1.8) -> (23.55, 1.8)
  line L27 (23.55, 1.8) -> (16.2, 1.8)
  line L28 (16.2, 1.8) -> (16.2, -1.8)
  line L29 (16.2, -1.8) -> (1.8, -1.8)
  line L30 (52.2, -16.8) -> (52.2, -9.3)
  line L31 (52.2, -9.3) -> (59.7, -9.3)
  line L32 (59.7, -9.3) -> (59.7, -16.8)
  line L33 (59.7, -16.8) -> (52.2, -16.8)
  line L34 (37.95, -16.8) -> (30.45, -16.8)
  line L35 (30.45, -16.8) -> (30.45, -9.3)
  line L36 (30.45, -9.3) -> (37.95, -9.3)
  line L37 (37.95, -9.3) -> (37.95, -16.8)
  circle A5 centre (0, -32) radius 1
  circle A6 centre (61.5, 0) radius 1
  circle A7 centre (0, 0) radius 1
  circle A8 centre (61.5, -32) radius 1
  line L38 (30.75, -29.2) -> (30.75, -25.2) construction
  line L39 (34.95, -27.2) -> (26.55, -27.2) construction
  circle A9 centre (30.75, -27.2) radius 1
extrude "Extrude13" cut sketch "sketch 9845" against normal blind 10 contours A5 | A6 | A7 | A8
sketch "Sketch20" plane through (0, 0, 21.4) normal (0, 0, -1) x (1, 0, 0)
  line L0 (62.0668, -135.2694) -> (69.9022, -135.362) construction
  line L1 (69.9022, -135.362) -> (69.9332, -132.7306) construction
  line L2 (69.9332, -132.7306) -> (62.0978, -132.638) construction
  line L3 (62.0978, -132.638) -> (62.0668, -135.2694) construction
  line L4 (83.5, -134) -> (92, -134)
  line L5 (83.8141, -135.2612) -> (91.6519, -135.3628) construction
  line L6 (91.6519, -135.3628) -> (91.6859, -132.7388) construction
  line L7 (91.6859, -132.7388) -> (83.8481, -132.6372) construction
  line L8 (83.8481, -132.6372) -> (83.8141, -135.2612) construction
  line L9 (40, -134) -> (48.5, -134)
  line L10 (40.3086, -135.2441) -> (48.1525, -135.3611) construction
  line L11 (48.1525, -135.3611) -> (48.1914, -132.7559) construction
  line L12 (48.1914, -132.7559) -> (40.3475, -132.6389) construction
  line L13 (40.3475, -132.6389) -> (40.3086, -135.2441) construction
  dimension "d108" = 0.8
  dimension "d112" = 0.8
  dimension "d114" = 0.8
  text T0 "OUT GND VCC" font "Arial" height 0.8 align left top in box 7.836 x 2.6316 at (62.0668, -135.2694) x (0.99993, -0.011806) y (0.011806, 0.99993) spacing 1 kerned
  text T1 "OUT GND VCC" font "Arial" height 0.8 align left top in box 7.8385 x 2.6242 at (83.8141, -135.2612) x (0.999916, -0.012956) y (0.012956, 0.999916) spacing 1 kerned
  text T2 "OUT GND VCC" font "Arial" height 0.8 align left top in box 7.8448 x 2.6055 at (40.3086, -135.2441) x (0.999889, -0.014915) y (0.014915, 0.999889) spacing 1 kerned
  constraint horizontal L4
  constraint midpoint L4
  constraint horizontal L9
  constraint midpoint L9
extrude "Extrude14" cut sketch "Sketch20" against normal blind 0.4 text T2 T0 T1
sketch "Sketch21" plane through (14, 0, 0) normal (-1, 0, 0) x (0, -1, 0)
  line L0 (-138.884, 26.4) -> (-130.884, 26.4)
  line L1 (-130.884, 26.4) -> (-130.884, 51.4)
  line L2 (-130.884, 51.4) -> (-138.884, 51.4)
  line L3 (-138.884, 51.4) -> (-138.884, 26.4)
  line L4 (-134.884, 26.4) -> (-134.884, 27.9)
  line L5 (-134.884, 27.9) -> (-134.884, 28.9) construction
  line L6 (-134.884, 28.9) -> (-134.884, 29.9) construction
  circle A0 centre (-134.884, 28.9) radius 1
  line L7 (-134.884, 29.9) -> (-134.884, 45.1) construction
  line L8 (-134.884, 37.5) -> (-133.884, 37.5) construction
  circle A1 centre (-134.884, 46.1) radius 1
  dimension "d121" = 1.5
  dimension "d122" = 1
  dimension "d123" = 1
  dimension "d124" = 2
  dimension "d125" = 15.2
  dimension "d126" = 1
  constraint midpoint L0 L4.start
  constraint perpendicular L0 L4
  constraint parallel L4 L5
  constraint parallel L5 L6
  constraint coincident L5.end L6.start
  constraint parallel L6 L7
  constraint midpoint L7 L8.start
  constraint perpendicular L7 L8
  constraint symmetric A0 L8 A1
  measures "d121" distance of L4.start L4.end
  measures "d122" distance of L4.end L5.end
  measures "d123" distance of L5.end L6.end
  measures "d124" diameter of A0
  measures "d125" distance of L6.end L7.end
  measures "d126" distance of L8.start L8.end
extrude "Extrude15" cut sketch "Sketch21" against normal blind 10 contours A0 | A1
mirror "Mirror5" about plane through (66, 134.884, 17.5) normal (1, 0, 0) of "Extrude15"
equation "d91 = 'BAT'"
equation "d109 = 'OUT GND VCC'"
equation "d113 = 'OUT GND VCC'"
equation "d115 = 'OUT GND VCC'"
